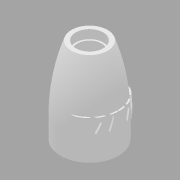
# Autodesk Inventor part: Lid
Saved by Autodesk Inventor 2019 (Build 230136000, 136)
## iProperties
Created: 2020-01-30
Part Number: Lid
Material: Generic
Document SubType Name: Modeling
Designer: alb16148
Density: 1 g/cm^3
Appearance: Default
Author: alb16148
Autodesk Inventor part; units mm, degrees
ref_plane "XZ Plane" through (0, 0, 0) normal (0, 1, 0) x (-1, 0, 0)
ref_plane "XY Plane" through (0, 0, 0) normal (0, 0, 1) x (1, 0, 0)
sketch "Sketch1" plane through (0, 0, 0) normal (1, 0, 0) x (0, 1, 0)
  line L0 (121, 3) -> (1, 3)
  line L1 (1, 3) -> (1, -3)
  line L2 (1, -3) -> (121, -3)
  line L3 (121, -3) -> (121, 3)
  line L4 (121, 3) -> (1, -3) construction
  line L5 (1, 3) -> (121, -3) construction
  line L6 (10, 8.35) -> (0, 8.35)
  line L7 (0, 8.35) -> (0, 20)
  line L8 (10, 8.35) -> (10, 9.45)
  line L9 (10, 9.45) -> (16, 9.45)
  line L10 (16, 9.45) -> (16, 17)
  line L11 (16, 17) -> (18, 17)
  line L12 (18, 17) -> (18, 18.5)
  line L13 (18, 18.5) -> (16, 18.5)
  line L14 (16, 18.5) -> (16, 20)
  line L15 (16, 20) -> (0, 20)
  line L16 (-24.2, 0) -> (145.2, 0) projected
  line L17 (16, 20) -> (31, 20)
  line L18 (18, 17) -> (31, 17)
  line L19 (75, 9.5) -> (69, 9.5)
  line L20 (69, 9.5) -> (69, 8.35)
  line L21 (69, 8.35) -> (66, 8.35)
  line L22 (75, 9.5) -> (75, 12.5)
  arc A0 (75, 12.5) -> (31, 20) centre (31, -112.8167) ccw
  arc A1 (59.0819, 13.9263) -> (31, 17) centre (31, -112.8167) ccw
  arc A2 (66, 8.35) -> (59.0819, 13.9263) centre (56.9187, 4.163) ccw
  point P0 (0, 0)
  point P1 (61, 0)
  point P2 (61, 0)
  dimension "d0" = 120
  dimension "d1" = 6
  dimension "d5" = 8.35
  dimension "d6" = 9.45
  dimension "d7" = 1.5
  dimension "d8" = 1.5
  dimension "d9" = 20
  dimension "d10" = 6
  dimension "d11" = 2
  dimension "d13" = 10
  dimension "d14" = 1
  dimension "d15" = 6
  dimension "d16" = 3
  dimension "d17" = 9.5
  dimension "d18" = 3
  dimension "d19" = 8.35
  dimension "d20" = 15
  dimension "d21" = 7.55
  dimension "d22" = 75
  dimension "d23" = 10
  constraints: 44 end point, 8 perpendicular, 7 horizontal, 6 point on circle, 3 centre point, 3 midpoint, 3 tangent, 3 vertical, 2 parallel, 2 vertical alignment, 1 collinear, 1 concentric, 1 horizontal alignment
  measures "d0" distance of L2.end L1.end
  measures "d1" distance of L1.end L0.end
  measures "d5" distance between parallel lines of L16 L6
  measures "d6" distance between parallel lines of L16 L9
  measures "d7" distance between parallel lines of L15 L13
  measures "d8" distance between parallel lines of L13 L11
  measures "d9" distance between parallel lines of L16 L15
  measures "d10" distance of L8.end L9.end
  measures "d11" distance of L12.end L13.end
  measures "d13" distance of L6.start L6.end
  measures "d14" distance from line of point (0, 0) L1
  measures "d15" distance of L19.start L19.end
  measures "d16" distance of L19.start L22.end
  measures "d17" distance between parallel lines of L16 L19
  measures "d18" distance of L20.end L21.end
  measures "d19" distance between parallel lines of L16 L21
  measures "d20" distance of L14.end L17.end
  measures "d21" distance of L9.end L10.end
  measures "d22" distance between parallel lines of L7 L22
  measures "d23" radius of A2
revolve "Revolution1" add sketch "Sketch1" angle 360 about axis through (0, -10, 0) along (0, 1, 0) contours L17 A0 L22 L19 L20 L21 A2 A1 L18 L12 L13 L14
ref_plane "Work Plane1" through (20, 0, 0) normal (1, 0, 0) x (0, 1, 0)
sketch "Sketch2" plane through (20, 0, 0) normal (1, 0, 0) x (0, 1, 0)
  line L0 (43.0702, 14.665) -> (43.0702, -13.7402) construction
  line L1 (43.0702, -13.7402) -> (5.5489, -13.7402) construction
  line L2 (5.5489, -13.7402) -> (5.5489, 14.665) construction
  line L3 (5.5489, 14.665) -> (43.0702, 14.665) construction
  line L4 (42.6848, 18.6603) -> (43.0598, 18.6812)
  line L5 (43.0598, 18.6812) -> (43.0286, 17.8166)
  spline S0 degree 2 poles (43.0286, 17.8166) (42.9869, 16.577) (42.9869, 16.2437) knots 0 0 0 1 1 1
  spline S1 degree 2 poles (42.9869, 16.2437) (42.9869, 15.1812) (43.0286, 14.6395) knots 0 0 0 1 1 1
  line L6 (43.0286, 14.6395) -> (43.0286, 13.9832)
  line L7 (43.0286, 13.9832) -> (42.6744, 13.9416)
  spline S2 degree 2 poles (42.6744, 13.9416) (42.6327, 14.4832) (42.2681, 15.452) (41.9348, 15.452) knots 0 0 0 1 2 2 2
  spline S3 degree 2 poles (41.9348, 15.452) (41.5806, 15.452) (37.5494, 14.0457) (33.3515, 12.4312) (33.2577, 12.3687) knots 0 0 0 1 2 3 3 3
  line L8 (33.2577, 12.3687) -> (34.2473, 11.9937)
  spline S4 degree 2 poles (34.2473, 11.9937) (34.3619, 11.9416) (35.539, 11.452) (35.8515, 11.327) knots 0 0 0 1 2 2 2
  line L9 (35.8515, 11.327) -> (39.4348, 9.7228)
  spline S5 degree 2 poles (39.4348, 9.7228) (41.0598, 10.4207) (41.9973, 10.8374) (42.1327, 10.9416) knots 0 0 0 1 2 2 2
  spline S6 degree 2 poles (42.1327, 10.9416) (42.6015, 11.2853) (42.6431, 11.9728) knots 0 0 0 1 1 1
  line L10 (42.6431, 11.9728) -> (43.0181, 12.0145)
  spline S7 degree 2 poles (43.0181, 12.0145) (42.9765, 11.3895) (42.9765, 10.7332) knots 0 0 0 1 1 1
  spline S8 degree 2 poles (42.9765, 10.7332) (42.9765, 9.0562) (43.0702, 7.7124) knots 0 0 0 1 1 1
  line L11 (43.0702, 7.7124) -> (42.7473, 7.6916)
  spline S9 degree 2 poles (42.7473, 7.6916) (42.6744, 8.3478) (42.414, 8.9728) (42.1431, 9.1082) (41.9452, 9.1082) knots 0 0 0 1 2 3 3 3
  spline S10 degree 2 poles (41.9452, 9.1082) (41.6327, 9.1082) (38.1327, 7.9416) (33.8098, 6.3166) (33.2265, 6.0562) knots 0 0 0 1 2 3 3 3
  spline S11 degree 2 poles (33.2265, 6.0562) (34.914, 5.3791) (38.6015, 4.0457) (41.164, 3.2645) (41.5494, 3.2645) knots 0 0 0 1 2 3 3 3
  spline S12 degree 2 poles (41.5494, 3.2645) (42.3098, 3.2645) (42.7056, 4.2957) (42.7369, 5.0457) knots 0 0 0 1 2 2 2
  line L12 (42.7369, 5.0457) -> (43.039, 5.1187)
  line L13 (43.039, 5.1187) -> (43.039, 4.1291)
  spline S13 degree 2 poles (43.039, 4.1291) (42.9973, 2.8999) (43.039, 1.3791) knots 0 0 0 1 1 1
  line L14 (43.039, 1.3791) -> (43.0598, 0.6395)
  line L15 (43.0598, 0.6395) -> (42.7369, 0.6707)
  spline S14 degree 2 poles (42.7369, 0.6707) (42.6848, 1.2437) (42.1848, 1.9832) (41.0077, 2.6291) (39.8723, 3.0457) knots 0 0 0 1 2 3 3 3
  line L16 (39.8723, 3.0457) -> (34.789, 4.8687)
  spline S15 degree 2 poles (34.789, 4.8687) (33.5494, 5.3374) (33.3306, 5.4207) knots 0 0 0 1 1 1
  spline S16 degree 2 poles (33.3306, 5.4207) (32.8723, 5.6082) (32.1744, 5.8478) (31.2473, 6.1603) (30.6431, 6.3687) knots 0 0 0 1 2 3 3 3
  line L17 (30.6431, 6.3687) -> (30.664, 6.6499)
  spline S17 degree 2 poles (30.664, 6.6499) (31.4348, 6.9103) (33.0598, 7.4207) (34.2265, 7.8166) (34.4869, 7.9207) knots 0 0 0 1 2 3 3 3
  line L18 (34.4869, 7.9207) -> (38.7369, 9.4728)
  spline S18 degree 2 poles (38.7369, 9.4728) (38.4556, 9.5978) (37.5806, 10.0041) (37.3619, 10.1187) knots 0 0 0 1 2 2 2
  line L19 (37.3619, 10.1187) -> (35.1536, 11.0874)
  spline S19 degree 2 poles (35.1536, 11.0874) (34.3306, 11.4624) (32.9452, 11.9728) (31.2681, 12.5353) (30.6431, 12.7332) knots 0 0 0 1 2 3 3 3
  line L20 (30.6431, 12.7332) -> (30.6431, 12.9832)
  line L21 (30.6431, 12.9832) -> (33.7473, 14.0666)
  spline S20 degree 2 poles (33.7473, 14.0666) (34.4556, 14.2957) (36.5494, 15.0041) (39.2473, 15.9624) (41.3098, 16.7645) (41.7265, 16.9937) knots 0 0 0 1 2 3 4 4 4
  spline S21 degree 2 poles (41.7265, 16.9937) (42.3515, 17.327) (42.6848, 18.1187) (42.6848, 18.6603) knots 0 0 0 1 2 2 2
  line L22 (42.6848, 0.1707) -> (43.0598, 0.1916)
  line L23 (43.0598, 0.1916) -> (43.0286, -0.673)
  spline S22 degree 2 poles (43.0286, -0.673) (42.9869, -1.9126) (42.9869, -2.2459) knots 0 0 0 1 1 1
  spline S23 degree 2 poles (42.9869, -2.2459) (42.9869, -3.3084) (43.0286, -3.8501) knots 0 0 0 1 1 1
  line L24 (43.0286, -3.8501) -> (43.0286, -4.5063)
  line L25 (43.0286, -4.5063) -> (42.6744, -4.548)
  spline S24 degree 2 poles (42.6744, -4.548) (42.6327, -4.0063) (42.2681, -3.0376) (41.9348, -3.0376) knots 0 0 0 1 2 2 2
  spline S25 degree 2 poles (41.9348, -3.0376) (41.5806, -3.0376) (37.5494, -4.4438) (33.3515, -6.0584) (33.2577, -6.1209) knots 0 0 0 1 2 3 3 3
  line L26 (33.2577, -6.1209) -> (34.2473, -6.4959)
  spline S26 degree 2 poles (34.2473, -6.4959) (34.3619, -6.548) (35.539, -7.0376) (35.8515, -7.1626) knots 0 0 0 1 2 2 2
  line L27 (35.8515, -7.1626) -> (39.4348, -8.7668)
  spline S27 degree 2 poles (39.4348, -8.7668) (41.0598, -8.0688) (41.9973, -7.6522) (42.1327, -7.548) knots 0 0 0 1 2 2 2
  spline S28 degree 2 poles (42.1327, -7.548) (42.6015, -7.2043) (42.6431, -6.5168) knots 0 0 0 1 1 1
  line L28 (42.6431, -6.5168) -> (43.0181, -6.4751)
  spline S29 degree 2 poles (43.0181, -6.4751) (42.9765, -7.1001) (42.9765, -7.7563) knots 0 0 0 1 1 1
  spline S30 degree 2 poles (42.9765, -7.7563) (42.9765, -9.4334) (43.0702, -10.7772) knots 0 0 0 1 1 1
  line L29 (43.0702, -10.7772) -> (42.7473, -10.798)
  spline S31 degree 2 poles (42.7473, -10.798) (42.6744, -10.1418) (42.414, -9.5168) (42.1431, -9.3813) (41.9452, -9.3813) knots 0 0 0 1 2 3 3 3
  spline S32 degree 2 poles (41.9452, -9.3813) (41.6327, -9.3813) (38.1327, -10.548) (33.8098, -12.173) (33.2265, -12.4334) knots 0 0 0 1 2 3 3 3
  spline S33 degree 2 poles (33.2265, -12.4334) (34.914, -13.1105) (38.6015, -14.4438) (41.164, -15.2251) (41.5494, -15.2251) knots 0 0 0 1 2 3 3 3
  spline S34 degree 2 poles (41.5494, -15.2251) (42.3098, -15.2251) (42.7056, -14.1938) (42.7369, -13.4438) knots 0 0 0 1 2 2 2
  line L30 (42.7369, -13.4438) -> (43.039, -13.3709)
  line L31 (43.039, -13.3709) -> (43.039, -14.3605)
  spline S35 degree 2 poles (43.039, -14.3605) (42.9973, -15.5897) (43.039, -17.1105) knots 0 0 0 1 1 1
  line L32 (43.039, -17.1105) -> (43.0598, -17.8501)
  line L33 (43.0598, -17.8501) -> (42.7369, -17.8188)
  spline S36 degree 2 poles (42.7369, -17.8188) (42.6848, -17.2459) (42.1848, -16.5063) (41.0077, -15.8605) (39.8723, -15.4438) knots 0 0 0 1 2 3 3 3
  line L34 (39.8723, -15.4438) -> (34.789, -13.6209)
  spline S37 degree 2 poles (34.789, -13.6209) (33.5494, -13.1522) (33.3306, -13.0688) knots 0 0 0 1 1 1
  spline S38 degree 2 poles (33.3306, -13.0688) (32.8723, -12.8813) (32.1744, -12.6418) (31.2473, -12.3293) (30.6431, -12.1209) knots 0 0 0 1 2 3 3 3
  line L35 (30.6431, -12.1209) -> (30.664, -11.8397)
  spline S39 degree 2 poles (30.664, -11.8397) (31.4348, -11.5793) (33.0598, -11.0688) (34.2265, -10.673) (34.4869, -10.5688) knots 0 0 0 1 2 3 3 3
  line L36 (34.4869, -10.5688) -> (38.7369, -9.0168)
  spline S40 degree 2 poles (38.7369, -9.0168) (38.4556, -8.8918) (37.5806, -8.4855) (37.3619, -8.3709) knots 0 0 0 1 2 2 2
  line L37 (37.3619, -8.3709) -> (35.1536, -7.4022)
  spline S41 degree 2 poles (35.1536, -7.4022) (34.3306, -7.0272) (32.9452, -6.5168) (31.2681, -5.9543) (30.6431, -5.7563) knots 0 0 0 1 2 3 3 3
  line L38 (30.6431, -5.7563) -> (30.6431, -5.5063)
  line L39 (30.6431, -5.5063) -> (33.7473, -4.423)
  spline S42 degree 2 poles (33.7473, -4.423) (34.4556, -4.1938) (36.5494, -3.4855) (39.2473, -2.5272) (41.3098, -1.7251) (41.7265, -1.4959) knots 0 0 0 1 2 3 4 4 4
  spline S43 degree 2 poles (41.7265, -1.4959) (42.3515, -1.1626) (42.6848, -0.3709) (42.6848, 0.1707) knots 0 0 0 1 2 2 2
  point P0 (0, 0)
  constraints: 2 other
emboss "Emboss1" sketch "Sketch2" operation add depth 1 direction (-1, 0, 0)
body "Solid1"
